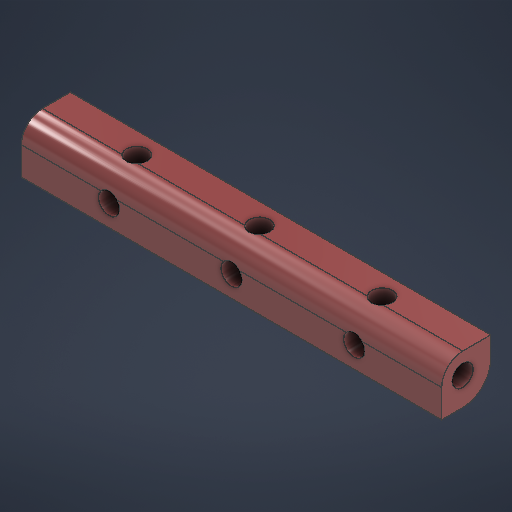
# Autodesk Inventor part: pillar
Saved by Autodesk Inventor 2026.1 (Build 301233000, 233)
## iProperties
Created: 2026-05-02
Part Number: pillar
Material: Generic
Document SubType Name: Modeling
Designer: emanuel
Density: 1 g/cm^3
Appearance: Default
Author: emanuel
Autodesk Inventor part; units mm, degrees
ref_plane "YZ Plane" through (0, 0, 0) normal (1, 0, 0) x (0, 1, 0)
ref_plane "XZ Plane" through (0, 0, 0) normal (0, 1, 0) x (-1, 0, 0)
ref_plane "XY Plane" through (0, 0, 0) normal (0, 0, 1) x (1, 0, 0)
sketch "Sketch1" plane through (0, 0, 0) normal (1, 0, 0) x (0, 1, 0)
  circle A0 centre (0, 0) radius 1.5
  circle A1 centre (0, 0) radius 3
  line L0 (0, 0) -> (-4, 0)
  line L1 (-4, 0) -> (-4, 3)
  line L2 (-4, 3) -> (0, 3)
  line L3 (0, 3) -> (0, 0)
  line L4 (0, 0) -> (3, 0)
  line L5 (3, 0) -> (3, -4)
  line L6 (3, -4) -> (0, -4)
  line L7 (0, -4) -> (0, 0)
  line L8 (0, 0) -> (-4, 0)
  line L9 (-4, 0) -> (-4, -4)
  line L10 (-4, -4) -> (0, -4)
  line L11 (0, -4) -> (0, 0)
  dimension "d0" = 3
  dimension "d1" = 6
  dimension "d2" = 4
  dimension "d3" = 4
  dimension "d6" = 4
  constraints: 24 end point, 6 parallel, 3 horizontal, 3 perpendicular, 2 centre point, 2 coincident, 1 point on line
  measures "d0" diameter of A0
  measures "d1" diameter of A1
  measures "d2" distance of L1.end L2.end
  measures "d3" distance of L4.end L5.end
  measures "d6" distance from line of L0.start L9
extrude "Extrusion1" add sketch "Sketch1" along normal blind 60 contours L4 A1 L7 A0 | A0 L3 A1 L4 | A0 L0 A1 L3 | L7 A1 L0 A0 | L5 L6 L7 A1 | A1 L0 L1 L2 | L7 L10 L9 L0 A1
fillet "Fillet1" radius 4 1 edges at (30, -4, -4)
sketch "Sketch2" plane through (0, 3, 0) normal (0, 1, 0) x (1, 0, 0)
  line L0 (0, 4) -> (60, 4) projected
  line L1 (30, 4) -> (30, 1)
  circle A0 centre (30, 1) radius 1.5
  point P0 (0, 0)
  dimension "d8" = 3
  dimension "d15" = 3
  constraints: 2 end point, 1 centre point, 1 coincident, 1 midpoint, 1 vertical
  measures "d8" diameter of A0
  measures "d15" distance of L1.start L1.end
extrude "Extrusion2" cut sketch "Sketch2" against normal blind 10
sketch "Sketch3" plane through (0, -4, 3) normal (0, 0, 1) x (1, 0, 0)
  line L0 (31.118, 0) -> (28.882, 0) projected
  line L1 (30, 0) -> (30, 3)
  circle A0 centre (30, 3) radius 1.5
  point P0 (0, 4)
  dimension "d11" = 3
  dimension "d12" = 3
  constraints: 2 end point, 1 centre point, 1 coincident, 1 midpoint, 1 vertical
  measures "d11" distance of L1.start L1.end
  measures "d12" diameter of A0
extrude "Extrusion3" cut sketch "Sketch3" against normal blind 10
sketch "Sketch4" plane through (0, 3, 0) normal (0, 1, 0) x (1, 0, 0)
  arc A0 (31.118, 0) -> (28.882, 0) centre (30, 1) ccw projected
  line L0 (12.5, 1) -> (47.5, 1)
  circle A1 centre (12.5, 1) radius 1.5
  circle A2 centre (47.5, 1) radius 1.5
  point P0 (0, 0)
  dimension "d16" = 35
  dimension "d17" = 3
  dimension "d18" = 3
  constraints: 2 centre point, 2 coincident, 2 end point, 1 horizontal, 1 midpoint
  measures "d16" distance of L0.start L0.end
  measures "d17" diameter of A1
  measures "d18" diameter of A2
extrude "Extrusion4" cut sketch "Sketch4" against normal blind 10 contours A1 | A2
sketch "Sketch5" plane through (0, -4, 3) normal (0, 0, 1) x (1, 0, 0)
  arc A0 (28.5423, 2.6464) -> (31.4577, 2.6464) centre (30, 3) ccw projected
  line L0 (12.5, 3) -> (47.5, 3)
  circle A1 centre (12.5, 3) radius 1.5
  circle A2 centre (47.5, 3) radius 1.5
  point P0 (0, 4)
  dimension "d21" = 35
  dimension "d22" = 3
  dimension "d23" = 3
  constraints: 2 centre point, 2 coincident, 2 end point, 1 horizontal, 1 midpoint
  measures "d21" distance of L0.start L0.end
  measures "d22" diameter of A1
  measures "d23" diameter of A2
extrude "Extrusion5" cut sketch "Sketch5" against normal blind 10
body "Solid1"
